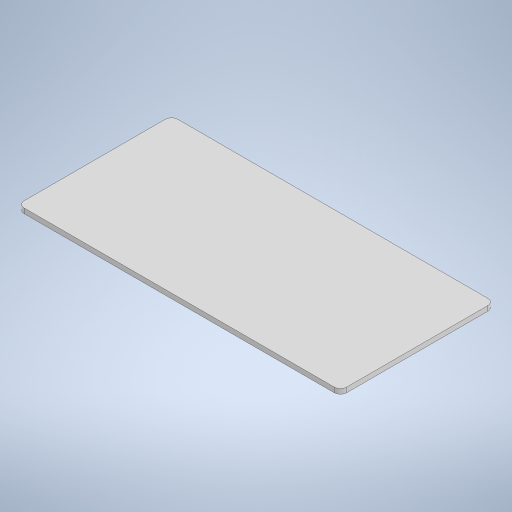
# Autodesk Inventor part: ty
Saved by Autodesk Inventor 2023 (Build 270158000, 158)
## iProperties
Created: 2024-03-30
Part Number: ty
Material: Ogólny
Document SubType Name: Modeling
Designer: Kamil
Density: 1 g/cm^3
Appearance: Domyślna
Author: Kamil
Autodesk Inventor part; units mm, degrees
ref_plane "YZ Plane" through (0, 0, 0) normal (1, 0, 0) x (0, 1, 0)
ref_plane "XZ Plane" through (0, 0, 0) normal (0, 1, 0) x (-1, 0, 0)
ref_plane "XY Plane" through (0, 0, 0) normal (0, 0, 1) x (1, 0, 0)
sketch "Szkic1" plane through (0, 0, 0) normal (0, 1, 0) x (-1, 0, 0)
  line L0 (52.5, 25) -> (-52.5, 25)
  line L1 (-52.5, 25) -> (-52.5, -25)
  line L2 (-52.5, -25) -> (52.5, -25)
  line L3 (52.5, -25) -> (52.5, 25)
  line L4 (52.5, 25) -> (-52.5, -25) construction
  line L5 (-52.5, 25) -> (52.5, -25) construction
  point P0 (0, 0)
  dimension "d0" = 105
  dimension "d1" = 50
  constraints: 12 end point, 2 midpoint, 2 parallel, 1 horizontal, 1 perpendicular
  measures "d0" distance of L1.end L2.end
  measures "d1" distance of L2.end L0.start
extrude "Wyciągnięcie proste1" add sketch "Szkic1" along normal blind 1.6
fillet "Zaokrąglenie1" radius 2 4 edges at (52.5, 0.8, 25) (52.5, 0.8, -25) (-52.5, 0.8, 25) (-52.5, 0.8, -25)
